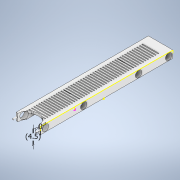
# Autodesk Inventor part: W-Link
Saved by Autodesk Inventor 2022.1 (Build 261234000, 234)
## iProperties
Company: El Camino College
Created: 2023-04-24
Part Number: W-Link
Material: PC/ABS Plastic
Document SubType Name: Modeling
Designer: Jerald Vanblaricom
Density: 0.357273 g/cm^3
Appearance: Smooth - White
Description: Left Side of the Bridge
Mass: 6.67211 g
Surface Area: 190.509 cm^2
Volume: 18.6751 cm^3
Author: Jerald Vanblaricom
Title: West Side Road
Autodesk Inventor part; units mm, degrees
ref_plane "YZ Plane" through (0, 0, 0) normal (1, 0, 0) x (0, 1, 0)
ref_plane "XZ Plane" through (0, 0, 0) normal (0, 1, 0) x (-1, 0, 0)
ref_plane "XY Plane" through (0, 0, 0) normal (0, 0, 1) x (1, 0, 0)
sketch "Sketch1" plane through (0, 0, 0) normal (0, 1, 0) x (-1, 0, 0)
  line L0 (-15, 77.5) -> (15, 77.5)
  line L1 (15, 77.5) -> (15, -77.5)
  line L2 (15, -77.5) -> (-15, -77.5)
  line L3 (-15, -77.5) -> (-15, 77.5)
  line L4 (-15, 77.5) -> (15, -77.5) construction
  line L5 (15, 77.5) -> (-15, -77.5) construction
  line L6 (-10, -75) -> (10, -75)
  line L7 (10, -75) -> (10, 75)
  line L8 (10, 75) -> (-10, 75)
  line L9 (-10, 75) -> (-10, -75)
  line L10 (-10, -75) -> (10, 75) construction
  line L11 (10, -75) -> (-10, 75) construction
  point P0 (0, 0)
  dimension "d0" = 30
  dimension "d1" = 155
  dimension "d2" = 20
  dimension "d3" = 150
  dimension "d4" = 2.5
  constraints: 24 end point, 4 midpoint, 4 parallel, 2 horizontal, 2 perpendicular
  measures "d0" distance of L1.end L2.end
  measures "d1" distance of L0.end L1.end
  measures "d2" distance of L8.end L7.end
  measures "d3" distance of L7.end L6.end
  measures "d4" distance between parallel lines of L0 L8
extrude "Extrusion1" add sketch "Sketch1" along normal blind 9
sketch "Sketch2" plane through (0, 9, 0) normal (0, 1, 0) x (1, 0, 0)
  line L0 (15, 77.5) -> (-15, 77.5) projected
  line L1 (-15, 77.5) -> (-15, -77.5) projected
  line L2 (-15, -77.5) -> (15, -77.5) projected
  line L3 (15, -77.5) -> (15, 77.5) projected
  line L4 (10, 75) -> (10, -75) projected
  line L5 (10, -75) -> (-10, -75) projected
  line L6 (-10, -75) -> (-10, 75) projected
  line L7 (-10, 75) -> (10, 75) projected
  line L8 (-10, -75) -> (-10, -73)
  line L9 (-10, -75) -> (-10, 75) projected
  line L10 (-10, -73) -> (10, -73)
  line L11 (10, 75) -> (10, -75) projected
  line L12 (10, -73) -> (10, -75)
  line L13 (10, -75) -> (-10, -75) projected
  line L14 (-10, -75) -> (10, -75)
  line L15 (-10, -71.98) -> (10, -71.98)
  line L16 (-10, -69.98) -> (10, -69.98)
  line L17 (-10, -71.98) -> (-10, -69.98)
  line L18 (10, -69.98) -> (10, -71.98)
  line L19 (-10, -68.96) -> (10, -68.96)
  line L20 (-10, -66.96) -> (10, -66.96)
  line L21 (-10, -68.96) -> (-10, -66.96)
  line L22 (10, -66.96) -> (10, -68.96)
  line L23 (-10, -65.94) -> (10, -65.94)
  line L24 (-10, -63.94) -> (10, -63.94)
  line L25 (-10, -65.94) -> (-10, -63.94)
  line L26 (10, -63.94) -> (10, -65.94)
  line L27 (-10, -62.92) -> (10, -62.92)
  line L28 (-10, -60.92) -> (10, -60.92)
  line L29 (-10, -62.92) -> (-10, -60.92)
  line L30 (10, -60.92) -> (10, -62.92)
  line L31 (-10, -59.9) -> (10, -59.9)
  line L32 (-10, -57.9) -> (10, -57.9)
  line L33 (-10, -59.9) -> (-10, -57.9)
  line L34 (10, -57.9) -> (10, -59.9)
  line L35 (-10, -56.88) -> (10, -56.88)
  line L36 (-10, -54.88) -> (10, -54.88)
  line L37 (-10, -56.88) -> (-10, -54.88)
  line L38 (10, -54.88) -> (10, -56.88)
  line L39 (-10, -53.86) -> (10, -53.86)
  line L40 (-10, -51.86) -> (10, -51.86)
  line L41 (-10, -53.86) -> (-10, -51.86)
  line L42 (10, -51.86) -> (10, -53.86)
  line L43 (-10, -50.84) -> (10, -50.84)
  line L44 (-10, -48.84) -> (10, -48.84)
  line L45 (-10, -50.84) -> (-10, -48.84)
  line L46 (10, -48.84) -> (10, -50.84)
  line L47 (-10, -47.82) -> (10, -47.82)
  line L48 (-10, -45.82) -> (10, -45.82)
  line L49 (-10, -47.82) -> (-10, -45.82)
  line L50 (10, -45.82) -> (10, -47.82)
  line L51 (-10, -44.8) -> (10, -44.8)
  line L52 (-10, -42.8) -> (10, -42.8)
  line L53 (-10, -44.8) -> (-10, -42.8)
  line L54 (10, -42.8) -> (10, -44.8)
  line L55 (-10, -41.78) -> (10, -41.78)
  line L56 (-10, -39.78) -> (10, -39.78)
  line L57 (-10, -41.78) -> (-10, -39.78)
  line L58 (10, -39.78) -> (10, -41.78)
  line L59 (-10, -38.76) -> (10, -38.76)
  line L60 (-10, -36.76) -> (10, -36.76)
  line L61 (-10, -38.76) -> (-10, -36.76)
  line L62 (10, -36.76) -> (10, -38.76)
  line L63 (-10, -35.74) -> (10, -35.74)
  line L64 (-10, -33.74) -> (10, -33.74)
  line L65 (-10, -35.74) -> (-10, -33.74)
  line L66 (10, -33.74) -> (10, -35.74)
  line L67 (-10, -32.72) -> (10, -32.72)
  line L68 (-10, -30.72) -> (10, -30.72)
  line L69 (-10, -32.72) -> (-10, -30.72)
  line L70 (10, -30.72) -> (10, -32.72)
  line L71 (-10, -29.7) -> (10, -29.7)
  line L72 (-10, -27.7) -> (10, -27.7)
  line L73 (-10, -29.7) -> (-10, -27.7)
  line L74 (10, -27.7) -> (10, -29.7)
  line L75 (-10, -26.68) -> (10, -26.68)
  line L76 (-10, -24.68) -> (10, -24.68)
  line L77 (-10, -26.68) -> (-10, -24.68)
  line L78 (10, -24.68) -> (10, -26.68)
  line L79 (-10, -23.66) -> (10, -23.66)
  line L80 (-10, -21.66) -> (10, -21.66)
  line L81 (-10, -23.66) -> (-10, -21.66)
  line L82 (10, -21.66) -> (10, -23.66)
  line L83 (-10, -20.64) -> (10, -20.64)
  line L84 (-10, -18.64) -> (10, -18.64)
  line L85 (-10, -20.64) -> (-10, -18.64)
  line L86 (10, -18.64) -> (10, -20.64)
  line L87 (-10, -17.62) -> (10, -17.62)
  line L88 (-10, -15.62) -> (10, -15.62)
  line L89 (-10, -17.62) -> (-10, -15.62)
  line L90 (10, -15.62) -> (10, -17.62)
  line L91 (-10, -14.6) -> (10, -14.6)
  line L92 (-10, -12.6) -> (10, -12.6)
  line L93 (-10, -14.6) -> (-10, -12.6)
  line L94 (10, -12.6) -> (10, -14.6)
  line L95 (-10, -11.58) -> (10, -11.58)
  line L96 (-10, -9.58) -> (10, -9.58)
  line L97 (-10, -11.58) -> (-10, -9.58)
  line L98 (10, -9.58) -> (10, -11.58)
  line L99 (-10, -8.56) -> (10, -8.56)
  line L100 (-10, -6.56) -> (10, -6.56)
  line L101 (-10, -8.56) -> (-10, -6.56)
  line L102 (10, -6.56) -> (10, -8.56)
  line L103 (-10, -5.54) -> (10, -5.54)
  line L104 (-10, -3.54) -> (10, -3.54)
  line L105 (-10, -5.54) -> (-10, -3.54)
  line L106 (10, -3.54) -> (10, -5.54)
  line L107 (-10, -2.52) -> (10, -2.52)
  line L108 (-10, -0.52) -> (10, -0.52)
  line L109 (-10, -2.52) -> (-10, -0.52)
  line L110 (10, -0.52) -> (10, -2.52)
  line L111 (-10, 0.5) -> (10, 0.5)
  line L112 (-10, 2.5) -> (10, 2.5)
  line L113 (-10, 0.5) -> (-10, 2.5)
  line L114 (10, 2.5) -> (10, 0.5)
  line L115 (-10, 3.52) -> (10, 3.52)
  line L116 (-10, 5.52) -> (10, 5.52)
  line L117 (-10, 3.52) -> (-10, 5.52)
  line L118 (10, 5.52) -> (10, 3.52)
  line L119 (-10, 6.54) -> (10, 6.54)
  line L120 (-10, 8.54) -> (10, 8.54)
  line L121 (-10, 6.54) -> (-10, 8.54)
  line L122 (10, 8.54) -> (10, 6.54)
  line L123 (-10, 9.56) -> (10, 9.56)
  line L124 (-10, 11.56) -> (10, 11.56)
  line L125 (-10, 9.56) -> (-10, 11.56)
  line L126 (10, 11.56) -> (10, 9.56)
  line L127 (-10, 12.58) -> (10, 12.58)
  line L128 (-10, 14.58) -> (10, 14.58)
  line L129 (-10, 12.58) -> (-10, 14.58)
  line L130 (10, 14.58) -> (10, 12.58)
  line L131 (-10, 15.6) -> (10, 15.6)
  line L132 (-10, 17.6) -> (10, 17.6)
  line L133 (-10, 15.6) -> (-10, 17.6)
  line L134 (10, 17.6) -> (10, 15.6)
  line L135 (-10, 18.62) -> (10, 18.62)
  line L136 (-10, 20.62) -> (10, 20.62)
  line L137 (-10, 18.62) -> (-10, 20.62)
  line L138 (10, 20.62) -> (10, 18.62)
  line L139 (-10, 21.64) -> (10, 21.64)
  line L140 (-10, 23.64) -> (10, 23.64)
  line L141 (-10, 21.64) -> (-10, 23.64)
  line L142 (10, 23.64) -> (10, 21.64)
  line L143 (-10, 24.66) -> (10, 24.66)
  line L144 (-10, 26.66) -> (10, 26.66)
  line L145 (-10, 24.66) -> (-10, 26.66)
  line L146 (10, 26.66) -> (10, 24.66)
  line L147 (-10, 27.68) -> (10, 27.68)
  line L148 (-10, 29.68) -> (10, 29.68)
  line L149 (-10, 27.68) -> (-10, 29.68)
  line L150 (10, 29.68) -> (10, 27.68)
  line L151 (-10, 30.7) -> (10, 30.7)
  line L152 (-10, 32.7) -> (10, 32.7)
  line L153 (-10, 30.7) -> (-10, 32.7)
  line L154 (10, 32.7) -> (10, 30.7)
  line L155 (-10, 33.72) -> (10, 33.72)
  line L156 (-10, 35.72) -> (10, 35.72)
  line L157 (-10, 33.72) -> (-10, 35.72)
  line L158 (10, 35.72) -> (10, 33.72)
  line L159 (-10, 36.74) -> (10, 36.74)
  line L160 (-10, 38.74) -> (10, 38.74)
  line L161 (-10, 36.74) -> (-10, 38.74)
  line L162 (10, 38.74) -> (10, 36.74)
  line L163 (-10, 39.76) -> (10, 39.76)
  line L164 (-10, 41.76) -> (10, 41.76)
  line L165 (-10, 39.76) -> (-10, 41.76)
  line L166 (10, 41.76) -> (10, 39.76)
  line L167 (-10, 42.78) -> (10, 42.78)
  line L168 (-10, 44.78) -> (10, 44.78)
  line L169 (-10, 42.78) -> (-10, 44.78)
  line L170 (10, 44.78) -> (10, 42.78)
  line L171 (-10, 45.8) -> (10, 45.8)
  line L172 (-10, 47.8) -> (10, 47.8)
  line L173 (-10, 45.8) -> (-10, 47.8)
  line L174 (10, 47.8) -> (10, 45.8)
  line L175 (-10, 48.82) -> (10, 48.82)
  line L176 (-10, 50.82) -> (10, 50.82)
  line L177 (-10, 48.82) -> (-10, 50.82)
  line L178 (10, 50.82) -> (10, 48.82)
  line L179 (-10, 51.84) -> (10, 51.84)
  line L180 (-10, 53.84) -> (10, 53.84)
  line L181 (-10, 51.84) -> (-10, 53.84)
  line L182 (10, 53.84) -> (10, 51.84)
  line L183 (-10, 54.86) -> (10, 54.86)
  line L184 (-10, 56.86) -> (10, 56.86)
  line L185 (-10, 54.86) -> (-10, 56.86)
  line L186 (10, 56.86) -> (10, 54.86)
  line L187 (-10, 57.88) -> (10, 57.88)
  line L188 (-10, 59.88) -> (10, 59.88)
  line L189 (-10, 57.88) -> (-10, 59.88)
  line L190 (10, 59.88) -> (10, 57.88)
  line L191 (-10, 60.9) -> (10, 60.9)
  line L192 (-10, 62.9) -> (10, 62.9)
  line L193 (-10, 60.9) -> (-10, 62.9)
  line L194 (10, 62.9) -> (10, 60.9)
  line L195 (-10, 63.92) -> (10, 63.92)
  line L196 (-10, 65.92) -> (10, 65.92)
  line L197 (-10, 63.92) -> (-10, 65.92)
  line L198 (10, 65.92) -> (10, 63.92)
  line L199 (-10, 66.94) -> (10, 66.94)
  line L200 (-10, 68.94) -> (10, 68.94)
  line L201 (-10, 66.94) -> (-10, 68.94)
  line L202 (10, 68.94) -> (10, 66.94)
  line L203 (-10, 70.14) -> (10, 70.14)
  line L204 (-10, 70.14) -> (-10, 72.14)
  line L205 (-10, 72.14) -> (10, 72.14)
  line L206 (10, 72.14) -> (10, 70.14)
  line L207 (-10, 73.34) -> (10, 73.34)
  line L208 (-10, 73.34) -> (-10, 75.34)
  line L209 (-10, 75.34) -> (10, 75.34)
  line L210 (10, 75.34) -> (10, 73.34)
  point P0 (0, 0)
  point P1 (10, 68.94)
  point P2 (-10, 68.94)
  point P3 (-10, 66.94)
  point P4 (10, 66.94)
  point P5 (10, 65.92)
  point P6 (-10, 65.92)
  point P7 (-10, 63.92)
  point P8 (10, 63.92)
  point P9 (10, 62.9)
  point P10 (-10, 62.9)
  point P11 (-10, 60.9)
  point P12 (10, 60.9)
  point P13 (10, 59.88)
  point P14 (-10, 59.88)
  point P15 (-10, 57.88)
  point P16 (10, 57.88)
  point P17 (10, 56.86)
  point P18 (-10, 56.86)
  point P19 (-10, 54.86)
  point P20 (10, 54.86)
  point P21 (10, 53.84)
  point P22 (-10, 53.84)
  point P23 (-10, 51.84)
  point P24 (10, 51.84)
  point P25 (10, 50.82)
  point P26 (-10, 50.82)
  point P27 (-10, 48.82)
  point P28 (10, 48.82)
  point P29 (10, 47.8)
  point P30 (-10, 47.8)
  point P31 (-10, 45.8)
  point P32 (10, 45.8)
  point P33 (10, 44.78)
  point P34 (-10, 44.78)
  point P35 (-10, 42.78)
  point P36 (10, 42.78)
  point P37 (10, 41.76)
  point P38 (-10, 41.76)
  point P39 (-10, 39.76)
  point P40 (10, 39.76)
  point P41 (10, 38.74)
  point P42 (-10, 38.74)
  point P43 (-10, 36.74)
  point P44 (10, 36.74)
  point P45 (10, 35.72)
  point P46 (-10, 35.72)
  point P47 (-10, 33.72)
  point P48 (10, 33.72)
  point P49 (10, 32.7)
  point P50 (-10, 32.7)
  point P51 (-10, 30.7)
  point P52 (10, 30.7)
  point P53 (10, 29.68)
  point P54 (-10, 29.68)
  point P55 (-10, 27.68)
  point P56 (10, 27.68)
  point P57 (10, 26.66)
  point P58 (-10, 26.66)
  point P59 (-10, 24.66)
  point P60 (10, 24.66)
  point P61 (10, 23.64)
  point P62 (-10, 23.64)
  point P63 (-10, 21.64)
  point P64 (10, 21.64)
  point P65 (10, 20.62)
  point P66 (-10, 20.62)
  point P67 (-10, 18.62)
  point P68 (10, 18.62)
  point P69 (10, 17.6)
  point P70 (-10, 17.6)
  point P71 (-10, 15.6)
  point P72 (10, 15.6)
  point P73 (10, 14.58)
  point P74 (-10, 14.58)
  point P75 (-10, 12.58)
  point P76 (10, 12.58)
  point P77 (10, 11.56)
  point P78 (-10, 11.56)
  point P79 (-10, 9.56)
  point P80 (10, 9.56)
  point P81 (10, 8.54)
  point P82 (-10, 8.54)
  point P83 (-10, 6.54)
  point P84 (10, 6.54)
  point P85 (10, 5.52)
  point P86 (-10, 5.52)
  point P87 (-10, 3.52)
  point P88 (10, 3.52)
  point P89 (10, 2.5)
  point P90 (-10, 2.5)
  point P91 (-10, 0.5)
  point P92 (10, 0.5)
  point P93 (10, -0.52)
  point P94 (-10, -0.52)
  point P95 (-10, -2.52)
  point P96 (10, -2.52)
  point P97 (10, -3.54)
  point P98 (-10, -3.54)
  point P99 (-10, -5.54)
  point P100 (10, -5.54)
  point P101 (10, -6.56)
  point P102 (-10, -6.56)
  point P103 (-10, -8.56)
  point P104 (10, -8.56)
  point P105 (10, -9.58)
  point P106 (-10, -9.58)
  point P107 (-10, -11.58)
  point P108 (10, -11.58)
  point P109 (10, -12.6)
  point P110 (-10, -12.6)
  point P111 (-10, -14.6)
  point P112 (10, -14.6)
  point P113 (10, -15.62)
  point P114 (-10, -15.62)
  point P115 (-10, -17.62)
  point P116 (10, -17.62)
  point P117 (10, -18.64)
  point P118 (-10, -18.64)
  point P119 (-10, -20.64)
  point P120 (10, -20.64)
  point P121 (10, -21.66)
  point P122 (-10, -21.66)
  point P123 (-10, -23.66)
  point P124 (10, -23.66)
  point P125 (10, -24.68)
  point P126 (-10, -24.68)
  point P127 (-10, -26.68)
  point P128 (10, -26.68)
  point P129 (10, -27.7)
  point P130 (-10, -27.7)
  point P131 (-10, -29.7)
  point P132 (10, -29.7)
  point P133 (10, -30.72)
  point P134 (-10, -30.72)
  point P135 (-10, -32.72)
  point P136 (10, -32.72)
  point P137 (10, -33.74)
  point P138 (-10, -33.74)
  point P139 (-10, -35.74)
  point P140 (10, -35.74)
  point P141 (10, -36.76)
  point P142 (-10, -36.76)
  point P143 (-10, -38.76)
  point P144 (10, -38.76)
  point P145 (10, -39.78)
  point P146 (-10, -39.78)
  point P147 (-10, -41.78)
  point P148 (10, -41.78)
  point P149 (10, -42.8)
  point P150 (-10, -42.8)
  point P151 (-10, -44.8)
  point P152 (10, -44.8)
  point P153 (10, -45.82)
  point P154 (-10, -45.82)
  point P155 (-10, -47.82)
  point P156 (10, -47.82)
  point P157 (10, -48.84)
  point P158 (-10, -48.84)
  point P159 (-10, -50.84)
  point P160 (10, -50.84)
  point P161 (10, -51.86)
  point P162 (-10, -51.86)
  point P163 (-10, -53.86)
  point P164 (10, -53.86)
  point P165 (10, -54.88)
  point P166 (-10, -54.88)
  point P167 (-10, -56.88)
  point P168 (10, -56.88)
  point P169 (10, -57.9)
  point P170 (-10, -57.9)
  point P171 (-10, -59.9)
  point P172 (10, -59.9)
  point P173 (10, -60.92)
  point P174 (-10, -60.92)
  point P175 (-10, -62.92)
  point P176 (10, -62.92)
  point P177 (10, -63.94)
  point P178 (-10, -63.94)
  point P179 (-10, -65.94)
  point P180 (10, -65.94)
  point P181 (-10, -66.96)
  point P182 (-10, -68.96)
  point P183 (10, -68.96)
  point P184 (-10, -69.98)
  point P185 (10, -71.98)
  point P186 (-10, 73.34)
  point P187 (10, 73.34)
  point P188 (10, 72.14)
  point P189 (-10, 72.14)
  point P190 (-10, 70.14)
  point P191 (10, 70.14)
  dimension "d7" = 2
  dimension "d10" = 3.02
  dimension "d67" = 3.2
  constraints: 400 end point, 196 vertical alignment, 98 collinear, 98 parallel, 2 horizontal, 2 point on line, 1 vertical
  measures "d7" distance of L5.end L8.end
  measures "d10" distance of L5.end L15.start
  measures "d67" distance of L199.start L203.start
extrude "Extrusion2" add sketch "Sketch2" against normal blind 3 contours L4 L207 L6 L7 | L7 L208 L209 L210 | L4 L203 L6 L205 | L4 L199 L6 L200 | L4 L195 L6 L196 | L4 L191 L6 L192 | L4 L187 L6 L188 | L4 L183 L6 L184 | L4 L179 L6 L180 | L4 L175 L6 L176 | L4 L171 L6 L172 | L4 L167 L6 L168 | L4 L163 L6 L164 | L4 L159 L6 L160 | L4 L155 L6 L156 | L4 L151 L6 L152 | L4 L147 L6 L148 | L4 L143 L6 L144 | L4 L139 L6 L140 | L4 L135 L6 L136 | L4 L131 L6 L132 | L4 L127 L6 L128 | L4 L123 L6 L124 | L4 L119 L6 L120 | L4 L115 L6 L116 | L4 L111 L6 L112 | L4 L107 L6 L108 | L4 L103 L6 L104 | L4 L99 L6 L100 | L4 L95 L6 L96 | L4 L91 L6 L92 | L4 L87 L6 L88 | L4 L83 L6 L84 | L4 L79 L6 L80 | L4 L75 L6 L76 | L4 L71 L6 L72 | L4 L67 L6 L68 | L4 L63 L6 L64 | L4 L59 L6 L60 | L4 L55 L6 L56 | L4 L51 L6 L52 | L4 L47 L6 L48 | L4 L43 L6 L44 | L4 L39 L6 L40 | L4 L35 L6 L36 | L4 L31 L6 L32 | L4 L27 L6 L28 | L4 L23 L6 L24 | L4 L19 L6 L20 | L4 L15 L6 L16 | L4 L5 L6 L10
sketch "Sketch3" plane through (15, 0, 77.5) normal (1, 0, 0) x (0, 0, -1)
  line L0 (155, 9) -> (0, 9) projected
  line L1 (0, 9) -> (5, 9)
  line L2 (5, 9) -> (5, 7.5)
  line L3 (155, 0) -> (0, 0) projected
  circle A0 centre (5, 7.5) radius 1
  line L4 (5, 9) -> (42.13, 9)
  line L5 (42.13, 9) -> (42.13, 7.5)
  line L6 (42.13, 9) -> (109.68, 9)
  line L7 (109.68, 9) -> (109.68, 7.5)
  line L8 (0, 9) -> (155, 9) projected
  line L9 (155, 0) -> (155, 9) projected
  line L10 (155, 9) -> (163, 9)
  line L11 (163, 9) -> (163, 6)
  line L12 (163, 6) -> (155, 6)
  line L13 (155, 6) -> (155, 9)
  point P0 (77.5, 0)
  dimension "d17" = 5
  dimension "d18" = 1.5
  dimension "d19" = 2
  dimension "d20" = 37.13
  dimension "d21" = 1.5
  dimension "d22" = 67.55
  dimension "d23" = 1.5
  dimension "d24" = 8
  constraints: 20 end point, 4 perpendicular, 3 point on line, 2 parallel, 1 centre point, 1 coincident, 1 horizontal
  measures "d17" distance of L0.end L1.end
  measures "d18" distance of L1.end L2.end
  measures "d19" diameter of A0
  measures "d20" distance of L1.end L4.end
  measures "d21" distance of L4.end L5.end
  measures "d22" distance of L4.end L6.end
  measures "d23" distance of L6.end L7.end
  measures "d24" distance of L11.end L12.end
extrude "Extrusion3" add sketch "Sketch3" against normal blind 16 contours L10 L11 L12 L9
sketch "Sketch5" plane through (15, 0, 77.5) normal (1, 0, 0) x (0, 0, -1)
  line L0 (0, 9) -> (163, 9) projected
  line L1 (0, 9) -> (0, 9)
  line L2 (0, 0) -> (0, 4.5)
  line L3 (0, 0) -> (0, 9) projected
  line L4 (163, 6) -> (163, 9) projected
  line L5 (41.76, 9) -> (41.76, 6) projected
  point P0 (77.5, 0)
  dimension "d38" = 0
  dimension "d39" = 4.5
  constraints: 4 end point, 1 midpoint, 1 point on line
  measures "d38" distance of L0.start L1.end
  measures "d39" distance of L2.start L2.end
sketch "Sketch7" plane through (15, 0, -77.5) normal (0, 0, -1) x (-1, 0, 0)
  line L0 (0, 0) -> (0, 6) projected
  line L1 (30, 0) -> (30, 9) projected
  line L2 (0, 0) -> (30, 0)
  line L3 (30, 0) -> (30, 9)
  line L4 (30, 9) -> (0, 9)
  line L5 (0, 9) -> (0, 0)
  line L6 (0, 9) -> (16, 9) projected
  point P0 (15, 0)
  point P1 (16, 6)
  constraints: 8 end point, 2 parallel, 1 collinear, 1 horizontal, 1 perpendicular, 2 other
extrude "Extrusion6" add sketch "Sketch7" along normal up to surface (8 mm away)
sketch "Sketch6" plane through (-15, 6, -85.5) normal (-1, 0, 0) x (0, 0, 1)
  line L0 (163, 3) -> (0, 3) projected
  line L1 (0, 3) -> (5, 3)
  line L2 (5, 3) -> (42.13, 3)
  line L3 (42.13, 3) -> (109.68, 3)
  line L4 (109.68, 3) -> (156.99, 3)
  circle A0 centre (156.99, -1.5) radius 4
  circle A1 centre (109.68, -1.5) radius 4
  circle A2 centre (42.13, -1.5) radius 4
  circle A3 centre (5, -1.5) radius 4
  line L5 (0, 0) -> (8, 0) projected
  line L6 (0, 3) -> (0, 0) projected
  point P0 (85.5, -6)
  dimension "d43" = 5
  dimension "d45" = 37.13
  dimension "d47" = 67.55
  dimension "d49" = 47.31
  dimension "d51" = 8
  dimension "d52" = 8
  dimension "d53" = 8
  dimension "d54" = 8
  dimension "d58" = 5
  dimension "d59" = 37.13
  dimension "d60" = 47.31
  dimension "d61" = 67.55
  constraints: 8 end point, 4 centre point, 4 point on line, 3 horizontal alignment
  measures "d43" distance of L0.end L1.end
  measures "d45" distance of L1.end L2.end
  measures "d47" distance of L2.end L3.end
  measures "d49" distance of L3.end L4.end
  measures "d51" diameter of A0
  measures "d52" diameter of A1
  measures "d53" diameter of A2
  measures "d54" diameter of A3
  measures "d58" distance from line of L6 A3.centre
  measures "d59" distance of A2.centre A3.centre
  measures "d60" distance of A0.centre A1.centre
  measures "d61" distance of A1.centre A2.centre
extrude "Insert_Holes" cut sketch "Sketch6" along normal through all both and the other way through all
sketch "Sketch12" plane through (0, 9, 0) normal (0, 1, 0) x (1, 0, 0)
  line L0 (-15, -77.5) -> (15, -77.5) projected
  circle A0 centre (0, -77.5) radius 12.7
  point P0 (0, 0)
  dimension "d84" = 25.4
  constraints: 1 centre point, 1 midpoint
  measures "d84" diameter of A0
extrude "Extrusion11" cut sketch "Sketch12" along normal through all both and the other way through all
sketch "Sketch13" plane through (15, 0, 77.5) normal (0, 0, 1) x (1, 0, 0)
  circle A0 centre (-1, 4.5) radius 0.75
  circle A1 centre (-29, 4.5) radius 0.75
  line L0 (0, 0) -> (0, 9) projected
  line L1 (-2.3, 0) -> (0, 0) projected
  line L2 (-30, 0) -> (-27.7, 0) projected
  line L3 (-30, 0) -> (-30, 9) projected
  point P0 (-15, 0)
  dimension "d87" = 1.5
  dimension "d88" = 1
  dimension "d89" = 4.5
  dimension "d90" = 4.5
  dimension "d91" = 1
  constraints: 2 centre point, 1 equal radius
  measures "d87" diameter of A0
  measures "d88" distance from line of L0 A0.centre
  measures "d89" distance from line of L1 A0.centre
  measures "d90" distance from line of L2 A1.centre
  measures "d91" distance from line of L3 A1.centre
extrude "Extrusion12" add sketch "Sketch13" along normal blind 5
body "Solid1"
